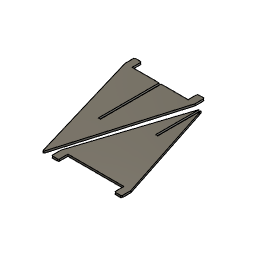
Gemüsehalter (Autodesk Fusion 360 design; units mm, degrees)
Autodesk Fusion 360 part; units mm, degrees
sketch "Skizze1" plane through (0, 0, 0) normal (0, 1, 0) x (1, 0, 0)
  line L0 (-60, 0) -> (0, 0)
  line L1 (0, 0) -> (0, -250)
  line L2 (0, -250) -> (-1, -250)
  line L3 (-1, -250) -> (-75, 0)
  line L4 (-75, 0) -> (-75, 20)
  line L5 (-75, 20) -> (-60, 20)
  line L6 (-60, 20) -> (-60, 0)
  line L7 (0, 0) -> (-2.2, 0)
  line L8 (-2.2, 0) -> (-2.2, -130)
  line L9 (-2.2, -130) -> (0, -130)
  line L10 (0, -130) -> (0, 0)
  line L11 (2.2, -130) -> (0, -130)
  line L12 (0, 0) -> (2.2, 0)
  line L13 (0, -250) -> (1, -250)
  line L14 (75, 0) -> (75, 20)
  line L15 (75, 20) -> (60, 20)
  line L16 (2.2, 0) -> (2.2, -130)
  line L17 (0, 0) -> (0, -250)
  line L18 (60, 20) -> (60, 0)
  line L19 (1, -250) -> (75, 0)
  line L20 (60, 0) -> (0, 0)
  line L21 (17.3489, -250) -> (17.3489, -230)
  line L22 (17.3489, -250) -> (32.3489, -250)
  line L23 (32.3489, -250) -> (32.3489, -230)
  line L24 (32.3489, -230) -> (92.3489, -230)
  line L25 (92.3489, -230) -> (92.3489, 0)
  line L26 (92.3489, 0) -> (17.3489, -230)
  line L27 (92.3489, -99.5) -> (90.1489, -99.5)
  line L28 (90.1489, -99.5) -> (90.1489, -6.7467)
  line L29 (92.3489, 0) -> (167.3489, -230)
  line L30 (167.3489, -250) -> (167.3489, -230)
  line L31 (167.3489, -250) -> (152.3489, -250)
  line L32 (152.3489, -250) -> (152.3489, -230)
  line L33 (152.3489, -230) -> (92.3489, -230)
  line L34 (94.5489, -99.5) -> (94.5489, -6.7467)
  line L35 (92.3489, -99.5) -> (94.5489, -99.5)
  dimension "d1" = 15
  dimension "d3" = 1
  dimension "d5" = 20
  dimension "d6" = 130
  dimension "d7" = 2.2
  dimension "d8" = 60
  dimension "d15" = 130.5
  dimension "d20" = 10
  dimension "d22" = 250
  constraint coincident L0.end L1.start
  constraint horizontal L0
  constraint perpendicular L0 L1
  constraint perpendicular L1 L2
  constraint perpendicular L2 L4
  constraint perpendicular L4 L5
  constraint perpendicular L0 L6
  constraint coincident L0 L3.end
  constraint horizontal L7
  constraint vertical L8
  constraint horizontal L9
  constraint vertical L10
  constraint symmetric L0.end L10 L1.start
  constraint symmetric L0.start L10 L18.end
  constraint symmetric L1.end L10 L2.start
  constraint symmetric L2.end L10 L13.end
  constraint symmetric L3.end L10 L14.start
  constraint symmetric L4.end L10 L14.end
  constraint symmetric L5.end L10 L15.end
  constraint symmetric L7.end L10 L12.end
  constraint symmetric L8.end L10 L11.start
  constraint symmetric L9.end L10 L11.end
  constraint parallel L17 L21
  constraint perpendicular L21 L22
  constraint perpendicular L22 L23
  constraint perpendicular L23 L24
  constraint perpendicular L24 L25
  constraint coincident L25 L27.start
  constraint perpendicular L25 L27
  constraint coincident L26 L28.end
  constraint perpendicular L27 L28
  constraint equal L9 L27
  constraint equal L6 L23
  constraint equal L0 L24
  constraint equal L4 L21
  constraint equal L5 L22
  constraint horizontal L0.end L25.end
  constraint symmetric L21.start L25 L30.start
  constraint symmetric L21.end L25 L29.end
  constraint symmetric L22.end L25 L31.end
  constraint symmetric L23.end L25 L32.end
  constraint symmetric L24.end L25 L33.end
  constraint symmetric L26.start L25 L29.start
  constraint symmetric L25 L27.start L35.start
  constraint symmetric L25 L27.end L34.start
  constraint symmetric L25 L28.end L34.end
  constraint collinear L13 L22
  measures "d1" distance of L4.end L5.end
  measures "d3" distance of L1.end L2.end
  measures "d5" distance of L0.end L5
  measures "d6" distance of L7.end L8.end
  measures "d7" distance of L1 L8
  measures "d8" distance of L0.start L0.end
  measures "d15" distance of L24 L27
  measures "d20" distance of L19 L21.end
  measures "d22" distance of L0.end L1.end
extrude "Extrusion1" add sketch "Skizze1" along normal blind 4 contours L0 L1 L2 L3 L4 L5 L6 L8 L9 L17 | L1 L11 L13 L14 L15 L16 L17 L18 L19 L20 | L21 L22 L23 L24 L25 L26 L27 L28 | L25 L29 L30 L31 L32 L33 L34 L35 makes body 1 at (-21.4667, 0, 43.3333) makes body 2 at (91.6155, 0, 186.5)
fillet "Abrundung1" radius 2 8 edges at (75, 2, -20) (60, 2, -20) (-60, 2, -20) (-75, 2, -20) (17.3489, 2, 250) (32.3489, 2, 250) (152.3489, 2, 250) (167.3489, 2, 250) on bodies 1 2
equation "d6 = d18 / 2"
equation "d15 = d6 + 0.5 mm"
equation "d18 = 260 mm"
